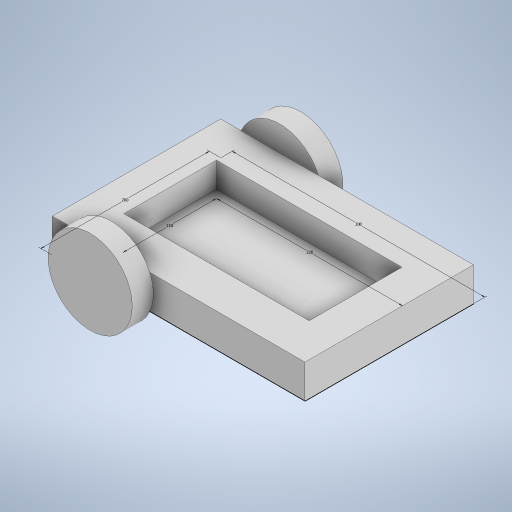
# Autodesk Inventor part: Chassis
Saved by Autodesk Inventor 2024 (Build 280153000, 153)
## iProperties
Created: 2023-07-03
Part Number: Chassis
Material: Generic
Document SubType Name: Modeling
Designer: janro
Density: 1 g/cm^3
Appearance: Default
Author: janro
Autodesk Inventor part; units mm, degrees
ref_plane "YZ Plane" through (0, 0, 0) normal (1, 0, 0) x (0, 1, 0)
ref_plane "XZ Plane" through (0, 0, 0) normal (0, 1, 0) x (-1, 0, 0)
ref_plane "XY Plane" through (0, 0, 0) normal (0, 0, 1) x (1, 0, 0)
sketch "Sketch1" plane through (0, 0, 0) normal (0, 1, 0) x (-1, 0, 0)
  line L0 (-110, 55) -> (110, 55)
  line L1 (110, 55) -> (110, -55)
  line L2 (110, -55) -> (-110, -55)
  line L3 (-110, -55) -> (-110, 55)
  line L4 (-110, 55) -> (110, -55) construction
  line L5 (110, 55) -> (-110, -55) construction
  line L6 (-150, 100) -> (150, 100)
  line L7 (150, 100) -> (150, -100)
  line L8 (150, -100) -> (-150, -100)
  line L9 (-150, -100) -> (-150, 100)
  line L10 (-150, 100) -> (150, -100) construction
  line L11 (150, 100) -> (-150, -100) construction
  point P0 (0, 0)
  dimension "d0" = 220
  dimension "d1" = 110
  dimension "d2" = 300
  dimension "d3" = 200
  constraints: 24 end point, 4 midpoint, 4 parallel, 2 horizontal, 2 perpendicular
  measures "d0" distance of L1.end L2.end
  measures "d1" distance of L0.end L1.end
  measures "d2" distance of L7.end L8.end
  measures "d3" distance of L6.end L7.end
extrude "Extrusion1" add sketch "Sketch1" along normal blind 10 contours L0 L1 L2 L3
extrude "Extrusion2" add sketch "Sketch1" along normal blind 40
sketch "Sketch2" plane through (-150, 0, 100) normal (0, 0, 1) x (1, 0, 0)
  line L0 (300, 0) -> (0, 0) projected
  line L1 (300, 0) -> (300, 40) projected
  line L2 (0, 0) -> (300, 0)
  line L3 (300, 0) -> (300, 40)
  line L4 (300, 40) -> (0, 40)
  line L5 (0, 40) -> (0, 0)
  circle A0 centre (70, 20) radius 50
  point P0 (150, 0)
  dimension "d8" = 100
  constraints: 8 end point, 2 parallel, 1 centre point, 1 horizontal, 1 perpendicular
  measures "d8" diameter of A0
sketch "Sketch3" plane through (150, 0, -100) normal (0, 0, -1) x (-1, 0, 0)
  line L0 (300, 0) -> (300, 40) projected
  line L1 (0, 40) -> (300, 40) projected
  line L2 (300, 0) -> (0, 0)
  line L3 (0, 0) -> (0, 40)
  line L4 (0, 40) -> (300, 40)
  line L5 (300, 40) -> (300, 0)
  line L6 (300, 0) -> (230, 0) construction
  line L7 (230, 0) -> (230, 20) construction
  line L8 (230, 20) -> (300, 20) construction
  line L9 (300, 20) -> (300, 0) construction
  circle A0 centre (230, 20) radius 50
  point P0 (150, 0)
  dimension "d9" = 70
  dimension "d10" = 20
  dimension "d11" = 100
  constraints: 16 end point, 4 parallel, 2 horizontal, 2 perpendicular, 1 centre point, 1 coincident
  measures "d9" distance of L7.end L8.end
  measures "d10" distance of L6.end L7.end
  measures "d11" diameter of A0
extrude "Extrusion3" add sketch "Sketch3" along normal blind 25 contours A0 L2 | L2 A0 L1 | L1 A0
extrude "Extrusion4" add sketch "Sketch2" along normal blind 25 contours A0 L0 | L0 A0 L4 | L4 A0
body "Solid1"
